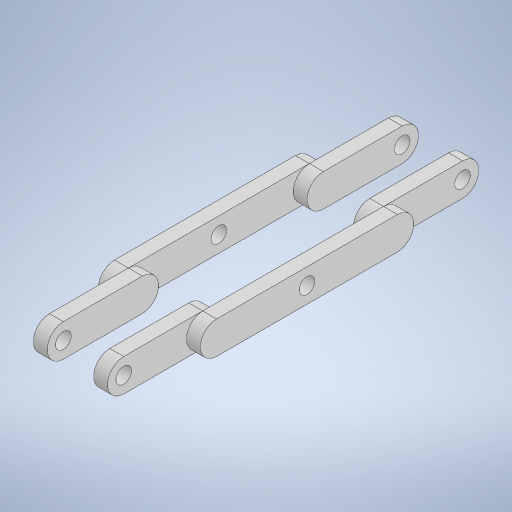
# Autodesk Inventor part: Corredera I
Saved by Autodesk Inventor 2024.3 (Build 283343000, 343)
## iProperties
Created: 2024-11-12
Part Number: Corredera I
Material: Generic
Document SubType Name: Modeling
Designer: j.santaa
Density: 1 g/cm^3
Appearance: Default
Author: j.santaa
Autodesk Inventor part; units mm, degrees
ref_plane "YZ Plane" through (0, 0, 0) normal (1, 0, 0) x (0, 1, 0)
ref_plane "XZ Plane" through (0, 0, 0) normal (0, 1, 0) x (-1, 0, 0)
ref_plane "XY Plane" through (0, 0, 0) normal (0, 0, 1) x (1, 0, 0)
sketch "Sketch1" plane through (0, 0, 0) normal (1, 0, 0) x (0, 1, 0)
  line L0 (0, -36.5) -> (0, 36.5) construction
  line L1 (3.5, -36.5) -> (3.5, 36.5)
  line L2 (-3.5, 36.5) -> (-3.5, -36.5)
  arc A0 (-3.5, -36.5) -> (3.5, -36.5) centre (0, -36.5) ccw
  arc A1 (3.5, 36.5) -> (-3.5, 36.5) centre (0, 36.5) ccw
  circle A2 centre (0, 36.5) radius 1.5
  circle A3 centre (0, 0) radius 1.5
  circle A4 centre (0, -36.5) radius 1.5
  line L3 (0, -19.5) -> (0, 19.5) construction
  line L4 (3.5, -19.5) -> (3.5, 19.5)
  line L5 (-3.5, 19.5) -> (-3.5, -19.5)
  arc A5 (-3.5, -19.5) -> (3.5, -19.5) centre (0, -19.5) ccw
  arc A6 (3.5, 19.5) -> (-3.5, 19.5) centre (0, 19.5) ccw
  line L6 (0, -36.5) -> (0, -19.5) construction
  line L7 (-3.5, -36.5) -> (-3.5, -19.5)
  line L8 (3.5, -19.5) -> (3.5, -36.5)
  arc A7 (-3.5, -36.5) -> (3.5, -36.5) centre (0, -36.5) ccw
  arc A8 (3.5, -19.5) -> (-3.5, -19.5) centre (0, -19.5) ccw
  line L9 (3.5, 0) -> (-3.5, 0) construction
  line L10 (0, 36.5) -> (0, 19.5) construction
  line L11 (-3.5, 36.5) -> (-3.5, 19.5)
  line L12 (3.5, 19.5) -> (3.5, 36.5)
  arc A9 (3.5, 36.5) -> (-3.5, 36.5) centre (0, 36.5) ccw
  arc A10 (-3.5, 19.5) -> (3.5, 19.5) centre (0, 19.5) ccw
  point P0 (0, -40)
  point P1 (0, 40)
  point P2 (3.5, 19.5)
  point P3 (-3.5, 19.5)
  point P4 (3.5, -19.5)
  point P5 (0, -28)
  point P6 (0, 28)
  point P7 (3.5, 19.5)
  point P8 (-3.5, 19.5)
  point P9 (-3.5, -19.5)
  point P10 (3.5, -19.5)
  dimension "d18" = 80
  dimension "d19" = 3
  dimension "d20" = 7
  dimension "d32" = 39
  constraints: 34 end point, 18 point on circle, 16 tangent, 11 centre point, 6 midpoint, 5 equal radius, 4 parallel, 3 coincident, 2 collinear, 1 point on line, 1 vertical
  measures "d18" distance of point (0, -40) point (0, 40)
  measures "d19" diameter of A3
  measures "d20" diameter of A1
  measures "d32" distance of L3.start L3.end
extrude "Extrusión3" add sketch "Sketch1" along normal mid plane 22 contours A8 L2 A10 L1 | A5 A8 | A10 A6 | A3
extrude "Extrusión4" cut sketch "Sketch1" along normal mid plane 16 contours A8 L2 A10 L1 | A5 A8 | A10 A6 | A3
extrude "Extrusión5" add sketch "Sketch1" along normal mid plane 16 contours A0 L2 A5 L1 | A5 A8 | A6 L2 A1 L1 | A10 A6 | A2 | A4
extrude "Extrusión6" cut sketch "Sketch1" along normal mid plane 10 contours A0 L2 A5 L1 | A5 A8 | A6 L2 A1 L1 | A10 A6 | A2 | A4
sketch "Boceto2" plane through (-8, 0, 0) normal (-1, 0, 0) x (0, 0, 1)
  point P0 (-36.5, 0)
  point P1 (36.5, 0)
hole "Agujero1" at (-8, 0, -36.5) at (-8, 0, 36.5) direction (1, 0, 0) diameter 3.4 end through all clearance for "Tornillo de cabeza plana avellanada ISO 2009/7046" size "M3" standard "ISO"
sketch "Boceto3" plane through (11, 0, 0) normal (1, 0, 0) x (0, 0, -1)
  point P0 (0, 0)
  point P1 (0, 0)
  constraints: 1 coincident
hole "Agujero2" at (11, 0, 0) direction (-1, 0, 0) diameter 3.4 end through all clearance for "Tornillo de cabeza plana avellanada ISO 2009/7046" size "M3" standard "ISO"
equation "\"d35\" = Dedos"
equation "\"Dedos\" = 10"
